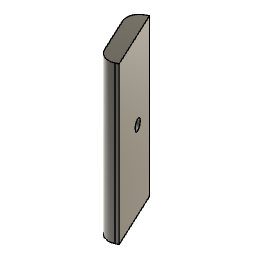
landing-gear-skid (Autodesk Fusion 360 design; units mm, degrees)
Autodesk Fusion 360 part; units mm, degrees
sketch "Sketch1" plane through (52.8799, 24.6583, 0) normal (-0.906308, -0.422618, 0) x (0.422618, -0.906308, 0)
  circle A0 centre (-1.1993, 6) radius 1
  line L0 (-5.8398, 0) -> (6.1602, 0)
  line L1 (6.1602, 0) -> (6.1602, 12) construction
  line L2 (6.1602, 12) -> (-5.8398, 12)
  line L3 (-5.8398, 12) -> (-5.8398, 0) construction
  line L4 (-5.8398, 21) -> (6.1602, 21)
  line L5 (6.1602, 21) -> (6.1602, -9)
  line L6 (6.1602, -9) -> (-5.8398, -9)
  line L7 (-5.8398, -9) -> (-5.8398, 21)
  line L8 (-5.8398, 0) -> (-5.8398, 12)
  line L9 (6.1602, 0) -> (6.1602, 12)
  line L10 (6.1602, 6) -> (-5.8398, 6) construction
  dimension "d27" = 15
  dimension "d29" = 30
  constraint horizontal L4
  constraint vertical L5
  constraint horizontal L6
  constraint vertical L7
  constraint coincident L4.end L9
  constraint coincident L2.end L7
  constraint midpoint L9 L10.start
  constraint midpoint L8 L10.end
  measures "d27" distance of L4 L10
  measures "d29" distance of L4 L6
extrude "Extrude1" add sketch "Sketch1" along normal blind 3
fillet "Fillet1" radius 2.4 2 edges at (47.693, 28.6831, 6) (52.7644, 17.8074, 6)
sketch "Sketch2" plane through (50.161, 23.3905, 0) normal (-0.906308, -0.422618, 0) x (0.422618, -0.906308, 0)
  circle A0 centre (-1.1993, 6) radius 1
  line L0 (3.7602, -9) -> (3.7602, 21)
  line L1 (3.7602, 21) -> (-3.4398, 21)
  line L2 (-3.4398, 21) -> (-3.4398, -9)
  line L3 (-3.4398, -9) -> (3.7602, -9)
  circle A1 centre (-1.1993, 6) radius 1
  circle A2 centre (-1.1993, 6) radius 1.5
  dimension "d34" = 3
  constraint concentric A1 A2
  measures "d34" diameter of A2
extrude "Extrude2" cut sketch "Sketch2" against normal blind 0.75 contours A0 A1 | A2
equation "d27 = skid_length / 2"
equation "d29 = skid_length"
equation "d30 = thickness"
equation "d33 = 0.8 * thickness"
equation "d35 = -thickness / 4"
equation "thickness = 3 mm"
equation "skid_length = 30 mm"
